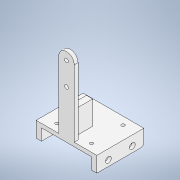
# Autodesk Inventor part: Support_batterie_réduit
Saved by Autodesk Inventor 2022 (Build 260153000, 153)
## iProperties
Created: 2021-12-07
Part Number: Support_batterie_réduit
Material: Générique
Document SubType Name: Modeling
Designer: utilisateur
Density: 1 g/cm^3
Appearance: Par défaut(1)
Author: utilisateur
Autodesk Inventor part; units mm, degrees
ref_plane "YZ Plane" through (0, 0, 0) normal (1, 0, 0) x (0, 1, 0)
ref_plane "XZ Plane" through (0, 0, 0) normal (0, 1, 0) x (-1, 0, 0)
ref_plane "XY Plane" through (0, 0, 0) normal (0, 0, 1) x (1, 0, 0)
sketch "Esquisse1" plane through (0, 0, 0) normal (0, 0, 1) x (1, 0, 0)
  line L0 (-10, 46) -> (10, 46) construction
  line L1 (10, 46) -> (10, -46)
  line L2 (10, -46) -> (-10, -46)
  line L3 (-10, -46) -> (-10, 46)
  line L4 (-10, 46) -> (10, -46) construction
  line L5 (10, 46) -> (-10, -46) construction
  arc A0 (10, 46) -> (-10, 46) centre (0, 46) ccw
  circle A1 centre (0, 46) radius 2.5
  line L6 (0, 46) -> (0, 16.2) construction
  circle A2 centre (0, 16.2) radius 2.5
  point P0 (0, 0)
  dimension "d0" = 29.8
  dimension "d1" = 5
  dimension "d2" = 20
  dimension "d3" = 92
  constraints: 14 end point, 3 centre point, 2 coincident, 2 midpoint, 2 parallel, 2 point on circle, 2 tangent, 1 equal radius, 1 horizontal, 1 perpendicular, 1 vertical
  measures "d0" distance of L6.start L6.end
  measures "d1" diameter of A1
  measures "d2" distance between parallel lines of L3 L1
  measures "d3" distance between parallel lines of L2 L0
extrude "Extrusion1" add sketch "Esquisse1" along normal blind 5
sketch "Esquisse2" plane through (-10, -46, 0) normal (0, -1, 0) x (1, 0, 0)
  line L0 (-22.4, -56) -> (-22.4, 5)
  line L1 (-22.4, 5) -> (42.4, 5)
  line L2 (42.4, 5) -> (42.4, -56)
  line L3 (42.4, -56) -> (-22.4, -56)
  line L4 (-22.4, -56) -> (42.4, 5) construction
  line L5 (-22.4, 5) -> (42.4, -56) construction
  line L6 (0, 5) -> (20, 5) projected
  line L7 (0, 5) -> (20, 5)
  line L8 (20, 0) -> (20, 5) projected
  line L9 (0, 0) -> (0, 5) projected
  line L10 (0, 0) -> (20, 0) projected
  line L11 (10, -25.5) -> (10, 0) construction
  line L12 (32.4, -46) -> (-12.4, -46) construction
  line L13 (-12.4, -46) -> (-12.4, -5) construction
  line L14 (-12.4, -5) -> (32.4, -5) construction
  line L15 (32.4, -5) -> (32.4, -46) construction
  line L16 (32.4, -46) -> (-12.4, -5) construction
  line L17 (-12.4, -46) -> (32.4, -5) construction
  circle A0 centre (-12.4, -46) radius 2.1
  circle A1 centre (32.4, -46) radius 2.1
  circle A2 centre (32.4, -5) radius 2.1
  circle A3 centre (-12.4, -5) radius 2.1
  line L18 (-22.4, 5) -> (-29.4, 5)
  line L19 (-29.4, 5) -> (-29.4, -56)
  line L20 (-29.4, -56) -> (-22.4, -56)
  line L21 (-22.4, -56) -> (-22.4, 5)
  line L22 (42.4, 5) -> (49.4, 5)
  line L23 (49.4, 5) -> (49.4, -56)
  line L24 (49.4, -56) -> (42.4, -56)
  line L25 (42.4, -56) -> (42.4, 5)
  dimension "d7" = 64.8
  dimension "d8" = 61
  dimension "d49" = 10
  dimension "d50" = 10
  dimension "d51" = 4.2
  dimension "d53" = 7
  constraints: 42 end point, 7 parallel, 5 horizontal, 4 centre point, 4 coincident, 4 midpoint, 3 collinear, 3 equal radius, 3 perpendicular, 3 vertical, 1 point on line, 3 other
  measures "d7" distance of L2.end L0.start
  measures "d8" distance of L2.start L2.end
  measures "d49" distance between parallel lines of L0 L13
  measures "d50" distance between parallel lines of L3 L12
  measures "d51" diameter of A3
  measures "d53" distance between parallel lines of L23 L2
extrude "Extrusion2" add sketch "Esquisse2" against normal blind 5
sketch "Esquisse10" plane through (0, 0, 0) normal (0, 0, -1) x (-1, 0, 0)
  line L0 (-4, -10.25) -> (4, -10.25)
  line L1 (4, -10.25) -> (4, -41)
  line L2 (4, -41) -> (-4, -41)
  line L3 (-4, -41) -> (-4, -10.25)
  line L4 (-4, -10.25) -> (4, -41) construction
  line L5 (4, -10.25) -> (-4, -41) construction
  line L6 (0, 0) -> (0, -25.625) construction
  line L7 (-4, -41) -> (4, -41)
  line L8 (4, -41) -> (4, -46)
  line L9 (4, -46) -> (-4, -46)
  line L10 (-4, -46) -> (-4, -41)
  line L11 (-10, -41) -> (10, -41) projected
  dimension "d41" = 8
  dimension "d48" = 30.75
  constraints: 22 end point, 4 parallel, 2 collinear, 2 horizontal, 2 midpoint, 2 perpendicular, 1 vertical
  measures "d41" distance between parallel lines of L3 L1
  measures "d48" distance of L0.end L1.end
extrude "Extrusion8" add sketch "Esquisse10" along normal blind 25
extrude "Extrusion10" add sketch "Esquisse2" along normal blind 15 contours L20 L19 L18 L0 | L2 L22 L23 L24
fillet "Congé2" radius 4 2 edges at (35.9, -61, -56) (-35.9, -61, -56)
sketch "Esquisse12" plane through (-39.4, -41, -56) normal (-1, 0, 0) x (0, 0, 1)
  arc A0 (0, -16) -> (4, -20) centre (4, -16) ccw projected
  line L0 (61, -20) -> (4, -20) projected
  line L1 (61, 0) -> (61, -20) projected
  line L2 (0, 0) -> (61, 0) projected
  line L3 (0, -16) -> (0, 0) projected
  line L4 (61, -5) -> (0, -5) projected
  line L5 (0, -5) -> (61, -5) projected
  line L6 (61, 0) -> (61, -20) projected
  line L7 (0, -5) -> (61, -5)
  line L8 (61, -5) -> (61, -20)
  line L9 (61, -20) -> (0, -20)
  line L10 (0, -20) -> (0, -5)
  line L11 (0, -5) -> (0, -16) projected
  line L12 (0, -12.5) -> (15, -12.5) construction
  line L13 (15, -12.5) -> (46, -12.5) construction
  line L14 (46, -12.5) -> (61, -12.5) construction
  circle A1 centre (15, -12.5) radius 2.05
  circle A2 centre (46, -12.5) radius 2.05
  circle A3 centre (15, -12.5) radius 3.75
  circle A4 centre (46, -12.5) radius 3.75
  point P0 (56, 41)
  dimension "d57" = 4.1
  dimension "d59" = 15
  dimension "d62" = 15
  dimension "d63" = 7.5
  constraints: 14 end point, 4 centre point, 4 coincident, 2 collinear, 2 equal radius, 2 parallel, 2 perpendicular, 2 point on line, 1 horizontal, 1 midpoint
  measures "d57" diameter of A2
  measures "d59" distance from line of L8 A2.centre
  measures "d62" distance between parallel lines of L9 L4
  measures "d63" diameter of A4
extrude "Extrusion11" cut sketch "Esquisse12" against normal through all contours A1 | A2
extrude "Extrusion12" cut sketch "Esquisse12" against normal blind 4 contours A3 | A4
sketch "Esquisse13" plane through (39.4, -41, 5) normal (1, 0, 0) x (0, 0, -1)
  circle A0 centre (46, -12.5) radius 3.75 projected
  circle A1 centre (15, -12.5) radius 3.75 projected
  point P0 (5, 41)
extrude "Extrusion13" cut sketch "Esquisse13" against normal blind 4
